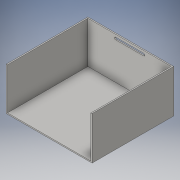
# Autodesk Inventor part: batteryholder-ver1-1111-2017
Saved by Autodesk Inventor 2016 SP1 (Build 200210100, 210)
## iProperties
Created: 2017-02-13
Part Number: batteryholder-ver1-1111-2017
Material: Generic
Document SubType Name: Modeling
Designer: 663531
Density: 1 g/cm^3
Appearance: Default
Author: 663531
Autodesk Inventor part; units mm, degrees
ref_plane "YZ Plane" through (0, 0, 0) normal (1, 0, 0) x (0, 1, 0)
ref_plane "XZ Plane" through (0, 0, 0) normal (0, 1, 0) x (-1, 0, 0)
ref_plane "XY Plane" through (0, 0, 0) normal (0, 0, 1) x (1, 0, 0)
sketch "Sketch1" plane through (0, 0, 0) normal (0, 0, 1) x (1, 0, 0)
  line L0 (0, 0) -> (-177.8, 0)
  line L1 (-177.8, 0) -> (-177.8, 88.9)
  line L2 (0, 0) -> (0, 88.9)
  line L3 (2.54, 88.9) -> (2.54, -2.54)
  line L4 (2.54, -2.54) -> (-180.34, -2.54)
  line L5 (-180.34, -2.54) -> (-180.34, 88.9)
  line L6 (-180.34, 88.9) -> (-177.8, 88.9)
  line L7 (2.54, 88.9) -> (0, 88.9)
  dimension "d0" = 177.8
  dimension "d2" = 2.54
  dimension "d13" = 88.9
  constraints: 16 end point, 2 horizontal, 2 perpendicular, 1 collinear, 1 parallel, 1 vertical, 2 other
  measures "d0" distance of L0.start L0.end
  measures "d2" distance between parallel lines of L2 L3
  measures "d13" distance between parallel lines of L6 L0
extrude "Extrusion1" add sketch "Sketch1" along normal blind 171.45
sketch "Sketch2" plane through (2.54, -2.54, 0) normal (1, 0, 0) x (0, 0, -1)
  line L0 (0, 0) -> (0, 91.44) projected
  line L1 (0, 0) -> (2.54, 0)
  line L2 (2.54, 0) -> (2.54, 91.44)
  line L3 (2.54, 91.44) -> (0, 91.44)
  line L4 (0, 91.44) -> (0, 0)
  point P0 (0, 2.54)
  point P1 (1.27, 91.44)
  dimension "d5" = 2.54
  constraints: 8 end point, 2 parallel, 1 horizontal, 1 horizontal alignment, 1 midpoint, 1 perpendicular
  measures "d5" distance of L3.end L2.end
extrude "Extrusion2" add sketch "Sketch2" against normal up to surface (182.88 mm away)
sketch "Sketch3" plane through (-177.8, 0, 0) normal (0, 0, 1) x (1, 0, 0)
  line L0 (56.6436, 81.28) -> (121.1564, 81.28) construction
  line L1 (59.1836, 78.74) -> (118.6164, 78.74)
  line L2 (118.6164, 83.82) -> (59.1836, 83.82)
  arc A0 (59.1836, 83.82) -> (59.1836, 78.74) centre (59.1836, 81.28) ccw
  arc A1 (118.6164, 78.74) -> (118.6164, 83.82) centre (118.6164, 81.28) ccw
  line L3 (177.8, 88.9) -> (0, 88.9) projected
  line L4 (177.8, 0) -> (0, 0) projected
  point P0 (88.9, 81.28)
  point P1 (88.9, 83.82)
  point P2 (88.9, 88.9)
  dimension "d9" = 5.08
  dimension "d10" = 81.28
  constraints: 8 end point, 6 point on circle, 4 tangent, 3 midpoint, 2 centre point, 2 point on line, 1 horizontal, 1 parallel, 1 vertical alignment
  measures "d9" diameter of A1
  measures "d10" distance from line of L4 point (88.9, 81.28)
extrude "Extrusion3" cut sketch "Sketch3" against normal through all
body "Solid1"
